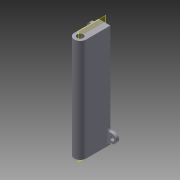
# Autodesk Inventor part: Pusher.Holder
Saved by Autodesk Inventor 2011 (Build 150239000, 239)
## iProperties
Created: 2011-04-01
Part Number: Pusher.Holder
Document SubType Name: Modeling
Designer: Rob
Density: 2.71 g/cm^3
Material: Aluminum-6061
Mass: 221.191 g
Surface Area: 204.196 cm^2
Volume: 81.6204 cm^3
Author: Rob
Autodesk Inventor part; units mm, degrees
note: some values were not read from the file. Chosen so that the rebuilt part matches the saved one: sketch regions of "Extrusion7".
ref_plane "YZ Plane" through (0, 0, 0) normal (1, 0, 0) x (0, 1, 0)
ref_plane "XZ Plane" through (0, 0, 0) normal (0, 1, 0) x (-1, 0, 0)
ref_plane "XY Plane" through (0, 0, 0) normal (0, 0, 1) x (1, 0, 0)
sketch "Sketch7" plane through (0, 0, 0) normal (0, 0, 1) x (1, 0, 0)
  circle A0 centre (0, 0) radius 4
  arc A1 (-8, 0) -> (8, 0) centre (0, 0) ccw
  line L0 (-8, 29) -> (-20, 29)
  line L1 (-20, 29) -> (-20, 33)
  line L2 (-20, 33) -> (0, 33)
  line L3 (0, 33) -> (20, 33)
  line L4 (20, 33) -> (20, 29)
  line L5 (20, 29) -> (8, 29)
  line L6 (-8, 0) -> (-8, 29)
  line L7 (8, 0) -> (8, 29)
  dimension "d34" = 4
  dimension "d35" = 33
  dimension "d36" = 8
  dimension "d37" = 4
  dimension "d38" = 12
  constraints: 16 end point, 4 perpendicular, 3 collinear, 2 centre point, 2 coincident, 2 parallel, 2 point on circle, 2 tangent, 1 horizontal
  measures "d34" distance of L0.end L1.end
  measures "d35" distance from line of L3 point (0, 0)
  measures "d36" diameter of A0
  measures "d37" radial gap between concentric circles of A1 A0
  measures "d38" distance of L0.start L0.end
extrude "Extrusion6" add sketch "Sketch7" along normal blind 140
sketch "Sketch8" plane through (-20, 29, 0) normal (0, -1, 0) x (1, 0, 0)
  line L0 (12, 140) -> (0, 140) projected
  line L1 (0, 0) -> (0, 140) projected
  line L2 (0, 0) -> (12, 0) projected
  line L3 (12, 0) -> (12, 140) projected
  line L4 (40, 140) -> (28, 140) projected
  line L5 (28, 0) -> (28, 140) projected
  line L6 (28, 0) -> (40, 0) projected
  line L7 (40, 0) -> (40, 140) projected
  line L8 (0, 134) -> (12, 134)
  line L9 (12, 134) -> (12, 122)
  line L10 (12, 122) -> (0, 122)
  line L11 (0, 122) -> (0, 134)
  line L12 (28, 6) -> (40, 6)
  line L13 (40, 6) -> (40, 18)
  line L14 (40, 18) -> (28, 18)
  line L15 (28, 18) -> (28, 6)
  point P0 (20, 0)
  dimension "d41" = 12
  dimension "d42" = 6
  dimension "d43" = 6
  constraints: 16 end point, 5 parallel, 4 point on line, 2 horizontal, 2 perpendicular
  measures "d41" distance between parallel lines of L14 L12
  measures "d42" distance between parallel lines of L12 L6
  measures "d43" distance between parallel lines of L8 L0
extrude "Extrusion7" cut sketch "Sketch8" against normal blind 140 contours L3 L8 L1 L0 | L3 L2 L1 L10 | L7 L14 L5 L4 | L7 L6 L5 L12
fillet "Fillet1" radius 6 4 edges at (20, 31, 6) (20, 31, 18) (-20, 31, 134) (-20, 31, 122)
fillet "Fillet1" radius 4 4 edges at (-8, 31, 134) (-8, 31, 122) (8, 31, 6) (8, 31, 18)
sketch "Sketch9" plane through (-14, 29, 122) normal (0, -1, 0) x (1, 0, 0)
  arc A0 (0, 12) -> (0, 0) centre (0, 6) ccw projected
  arc A1 (28, -116) -> (28, -104) centre (28, -110) ccw projected
  line L0 (28, -104) -> (26, -104) projected
  arc A2 (22, -100) -> (26, -104) centre (26, -100) ccw projected
  line L1 (22, -120) -> (22, -100) projected
  arc A3 (26, -116) -> (22, -120) centre (26, -120) ccw projected
  line L2 (26, -116) -> (28, -116) projected
  point P0 (14, -122)
hole "Hole2" at (14, 29, 12) at (-14, 29, 128) direction (0, 1, 0) diameter 6 depth 8 tip angle 118 clearance for "Flat Head Machine Screw" size "M6" standard "Ansi Metric M Profile"
sketch "Sketch10" plane through (0, 0, 140) normal (0, 0, 1) x (1, 0, 0)
  arc A0 (-8, 0) -> (8, 0) centre (0, 0) ccw projected
hole "Hole3" at (0, 0, 140) direction (0, 0, -1) diameter 8.376 depth 20 tip angle 118 thread size "M10x1.5" class "6H" standard "ANSI Metric M Profile"
sketch "Sketch11" plane through (0, 0, 0) normal (0, 0, -1) x (-1, 0, 0)
  arc A0 (-8, 0) -> (8, 0) centre (0, 0) ccw projected
hole "Hole4" at (0, 0, 0) direction (0, 0, 1) diameter 8.376 depth 20 tip angle 118 thread size "M10x1.5" class "6H" standard "ANSI Metric M Profile"
ref_plane "Work Plane3" through (0, 0, 140) normal (1, 0, 0) x (0, 0, -1)
body "Solid1"
body "Solid2"
